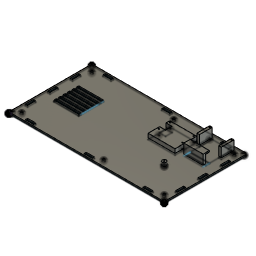
GBS 8200 Unterteil v2 (Autodesk Fusion 360 design; units mm, degrees)
Autodesk Fusion 360 part; units mm, degrees
sketch "Skizze1" plane through (0, 0, 0) normal (0, 1, 0) x (1, 0, 0)
  line L0 (2, 0) -> (206, 0)
  line L1 (208, 2) -> (208, 109)
  line L2 (206, 111) -> (2, 111)
  line L3 (0, 109) -> (0, 2)
  circle A0 centre (8.575, 8.575) radius 1.5
  circle A1 centre (8.575, 102.425) radius 1.5
  circle A2 centre (199.425, 102.425) radius 1.5
  circle A3 centre (199.425, 8.575) radius 1.5
  circle A4 centre (118.425, 8.575) radius 1.5
  circle A5 centre (118.425, 102.425) radius 1.5
  line L4 (123.425, 92.03) -> (159.425, 92.03)
  line L5 (159.425, 92.03) -> (159.425, 63.03)
  line L6 (159.425, 63.03) -> (123.425, 63.03)
  line L7 (123.425, 63.03) -> (123.425, 92.03)
  line L8 (123.425, 87.03) -> (131.425, 87.03)
  line L9 (131.425, 87.03) -> (131.425, 78.33)
  line L10 (131.425, 78.33) -> (123.425, 78.33)
  line L11 (123.425, 78.33) -> (123.425, 87.03)
  circle A6 centre (125.525, 90.23) radius 0.8
  circle A7 centre (157.325, 90.23) radius 0.8
  circle A8 centre (157.325, 75.23) radius 0.8
  circle A9 centre (125.525, 75.23) radius 0.8
  circle A10 centre (165.425, 42.575) radius 2.7
  circle A11 centre (165.425, 42.575) radius 0.8
  line L12 (166.2, 106) -> (192, 106)
  line L13 (192, 106) -> (192, 71.4)
  line L14 (192, 71.4) -> (166.2, 71.4)
  line L15 (166.2, 71.4) -> (166.2, 106)
  line L16 (166.2, 106) -> (162.8, 106)
  line L17 (162.8, 106) -> (162.8, 89)
  line L18 (162.8, 89) -> (166.2, 89)
  line L19 (166.2, 89) -> (166.2, 106)
  line L20 (192, 106) -> (195.4, 106)
  line L21 (195.4, 106) -> (195.4, 89)
  line L22 (195.4, 89) -> (192, 89)
  line L23 (192, 89) -> (192, 106)
  circle A12 centre (164.5, 104.3) radius 0.8
  circle A13 centre (193.7, 104.3) radius 0.8
  line L24 (166.2, 68) -> (192, 68)
  line L25 (192, 68) -> (192, 76.4)
  line L26 (192, 76.4) -> (166.2, 76.4)
  line L27 (166.2, 76.4) -> (166.2, 68)
  line L28 (166.2, 76.4) -> (192, 76.4)
  line L29 (192, 76.4) -> (192, 71.4)
  line L30 (192, 71.4) -> (166.2, 71.4)
  line L31 (166.2, 71.4) -> (166.2, 76.4)
  line L32 (16.5, 77) -> (49.5, 77)
  line L33 (49.5, 77) -> (49.5, 44)
  line L34 (49.5, 44) -> (16.5, 44)
  line L35 (16.5, 44) -> (16.5, 77)
  line L36 (16.5, 77) -> (49.5, 77)
  line L37 (49.5, 77) -> (49.5, 74)
  line L38 (49.5, 74) -> (16.5, 74)
  line L39 (16.5, 74) -> (16.5, 77)
  line L40 (16.5, 74) -> (49.5, 74)
  line L41 (49.5, 74) -> (49.5, 71)
  line L42 (49.5, 71) -> (16.5, 71)
  line L43 (16.5, 71) -> (16.5, 74)
  line L44 (16.5, 71) -> (49.5, 71)
  line L45 (49.5, 71) -> (49.5, 68)
  line L46 (49.5, 68) -> (16.5, 68)
  line L47 (16.5, 68) -> (16.5, 71)
  line L48 (16.5, 68) -> (49.5, 68)
  line L49 (49.5, 68) -> (49.5, 65)
  line L50 (49.5, 65) -> (16.5, 65)
  line L51 (16.5, 65) -> (16.5, 68)
  line L52 (16.5, 65) -> (49.5, 65)
  line L53 (49.5, 65) -> (49.5, 62)
  line L54 (49.5, 62) -> (16.5, 62)
  line L55 (16.5, 62) -> (16.5, 65)
  line L56 (16.5, 62) -> (49.5, 62)
  line L57 (49.5, 62) -> (49.5, 59)
  line L58 (49.5, 59) -> (16.5, 59)
  line L59 (16.5, 59) -> (16.5, 62)
  line L60 (16.5, 59) -> (49.5, 59)
  line L61 (49.5, 59) -> (49.5, 56)
  line L62 (49.5, 56) -> (16.5, 56)
  line L63 (16.5, 56) -> (16.5, 59)
  line L64 (16.5, 56) -> (49.5, 56)
  line L65 (49.5, 56) -> (49.5, 53)
  line L66 (49.5, 53) -> (16.5, 53)
  line L67 (16.5, 53) -> (16.5, 56)
  line L68 (16.5, 53) -> (49.5, 53)
  line L69 (49.5, 53) -> (49.5, 50)
  line L70 (49.5, 50) -> (16.5, 50)
  line L71 (16.5, 50) -> (16.5, 53)
  line L72 (16.5, 50) -> (49.5, 50)
  line L73 (49.5, 50) -> (49.5, 47)
  line L74 (49.5, 47) -> (16.5, 47)
  line L75 (16.5, 47) -> (16.5, 50)
  line L76 (16.5, 47) -> (49.5, 47)
  line L77 (49.5, 47) -> (49.5, 44)
  line L78 (49.5, 44) -> (16.5, 44)
  line L79 (16.5, 44) -> (16.5, 47)
  line L80 (20, 109) -> (30.8, 109)
  line L81 (30.8, 109) -> (30.8, 106)
  line L82 (30.8, 106) -> (20, 106)
  line L83 (20, 106) -> (20, 109)
  line L84 (2, 91) -> (5, 91)
  line L85 (5, 91) -> (5, 80.2)
  line L86 (5, 80.2) -> (2, 80.2)
  line L87 (2, 80.2) -> (2, 91)
  line L88 (2, 30.8) -> (5, 30.8)
  line L89 (5, 30.8) -> (5, 20)
  line L90 (5, 20) -> (2, 20)
  line L91 (2, 20) -> (2, 30.8)
  line L92 (20, 5) -> (30.8, 5)
  line L93 (30.8, 5) -> (30.8, 2)
  line L94 (30.8, 2) -> (20, 2)
  line L95 (20, 2) -> (20, 5)
  line L96 (177.2, 5) -> (188, 5)
  line L97 (188, 5) -> (188, 2)
  line L98 (188, 2) -> (177.2, 2)
  line L99 (177.2, 2) -> (177.2, 5)
  line L100 (203, 30.8) -> (206, 30.8)
  line L101 (206, 30.8) -> (206, 20)
  line L102 (206, 20) -> (203, 20)
  line L103 (203, 20) -> (203, 30.8)
  line L104 (177.2, 109) -> (188, 109)
  line L105 (188, 109) -> (188, 106)
  line L106 (188, 106) -> (177.2, 106)
  line L107 (177.2, 106) -> (177.2, 109)
  line L108 (203, 91) -> (206, 91)
  line L109 (206, 91) -> (206, 80.2)
  line L110 (206, 80.2) -> (203, 80.2)
  line L111 (203, 80.2) -> (203, 91)
  line L112 (98.6, 5) -> (109.4, 5)
  line L113 (109.4, 5) -> (109.4, 2)
  line L114 (109.4, 2) -> (98.6, 2)
  line L115 (98.6, 2) -> (98.6, 5)
  line L116 (98.6, 109) -> (109.4, 109)
  line L117 (109.4, 109) -> (109.4, 106)
  line L118 (109.4, 106) -> (98.6, 106)
  line L119 (98.6, 106) -> (98.6, 109)
  line L120 (203, 60.9) -> (206, 60.9)
  line L121 (206, 60.9) -> (206, 50.1)
  line L122 (206, 50.1) -> (203, 50.1)
  line L123 (203, 50.1) -> (203, 60.9)
  line L124 (2, 60.9) -> (5, 60.9)
  line L125 (5, 60.9) -> (5, 50.1)
  line L126 (5, 50.1) -> (2, 50.1)
  line L127 (2, 50.1) -> (2, 60.9)
  arc A14 (2, 111) -> (0, 109) centre (2, 109) ccw
  arc A15 (0, 2) -> (2, 0) centre (2, 2) ccw
  arc A16 (206, 0) -> (208, 2) centre (206, 2) ccw
  arc A17 (208, 109) -> (206, 111) centre (206, 109) ccw
  point P0 (208, 0)
  point P1 (0, 111)
  dimension "d1" = 208
  dimension "d2" = 111
  dimension "d3" = 3
  dimension "d4" = 8.575
  dimension "d5" = 8.575
  dimension "d6" = 3
  dimension "d7" = 8.575
  dimension "d8" = 8.575
  dimension "d9" = 3
  dimension "d10" = 8.575
  dimension "d11" = 8.575
  dimension "d12" = 3
  dimension "d13" = 8.575
  dimension "d14" = 8.575
  dimension "d15" = 3
  dimension "d16" = 8.575
  dimension "d17" = 109.85
  dimension "d18" = 3
  dimension "d19" = 8.575
  dimension "d20" = 109.85
  dimension "d21" = 36
  dimension "d22" = 29
  dimension "d23" = 18.97
  dimension "d24" = 5
  dimension "d25" = 5
  dimension "d26" = 8.7
  dimension "d27" = 8
  dimension "d28" = 1.6
  dimension "d29" = 1.6
  dimension "d30" = 31.8
  dimension "d31" = 2.1
  dimension "d32" = 1.8
  dimension "d33" = 1.8
  dimension "d34" = 1.6
  dimension "d35" = 2.1
  dimension "d36" = 15
  dimension "d37" = 1.6
  dimension "d38" = 15
  dimension "d39" = 2.1
  dimension "d40" = 5.4
  dimension "d41" = 34
  dimension "d42" = 34
  dimension "d43" = 1.6
  dimension "d44" = 25.8
  dimension "d45" = 34.6
  dimension "d46" = 5
  dimension "d47" = 16
  dimension "d48" = 3.4
  dimension "d49" = 3.4
  dimension "d50" = 17
  dimension "d51" = 17
  dimension "d52" = 1.6
  dimension "d53" = 1.7
  dimension "d54" = 1.7
  dimension "d55" = 1.6
  dimension "d56" = 1.7
  dimension "d57" = 1.7
  dimension "d58" = 8.4
  dimension "d59" = 5
  dimension "d60" = 33
  dimension "d61" = 33
  dimension "d62" = 34
  dimension "d63" = 16.5
  dimension "d64" = 3
  dimension "d65" = 33
  dimension "d66" = 3
  dimension "d67" = 3
  dimension "d68" = 3
  dimension "d69" = 3
  dimension "d70" = 3
  dimension "d71" = 3
  dimension "d72" = 3
  dimension "d73" = 3
  dimension "d74" = 3
  dimension "d75" = 10.8
  dimension "d76" = 3
  dimension "d77" = 20
  dimension "d78" = 2
  dimension "d79" = 3
  dimension "d80" = 10.8
  dimension "d81" = 2
  dimension "d82" = 20
  dimension "d83" = 3
  dimension "d84" = 10.8
  dimension "d85" = 2
  dimension "d86" = 20
  dimension "d87" = 10.8
  dimension "d88" = 3
  dimension "d89" = 2
  dimension "d90" = 20
  dimension "d91" = 10.8
  dimension "d92" = 3
  dimension "d93" = 2
  dimension "d94" = 20
  dimension "d95" = 3
  dimension "d96" = 10.8
  dimension "d97" = 2
  dimension "d98" = 20
  dimension "d99" = 10.8
  dimension "d100" = 3
  dimension "d101" = 2
  dimension "d102" = 20
  dimension "d103" = 3
  dimension "d104" = 10.8
  dimension "d105" = 2
  dimension "d106" = 20
  dimension "d107" = 10.8
  dimension "d108" = 3
  dimension "d109" = 2
  dimension "d110" = 98.6
  dimension "d111" = 10.8
  dimension "d112" = 3
  dimension "d113" = 2
  dimension "d114" = 98.6
  dimension "d115" = 3
  dimension "d116" = 10.8
  dimension "d117" = 2
  dimension "d118" = 50.1
  dimension "d119" = 3
  dimension "d120" = 10.8
  dimension "d121" = 2
  dimension "d122" = 50.1
  dimension "d123" = 2
  dimension "d124" = 2
  dimension "d125" = 2
  dimension "d126" = 2
  constraint horizontal L0
  constraint vertical L1
  constraint horizontal L2
  constraint vertical L3
  constraint horizontal L4
  constraint vertical L5
  constraint horizontal L6
  constraint vertical L7
  constraint horizontal L8
  constraint vertical L9
  constraint horizontal L10
  constraint vertical L11
  constraint coincident L7 L8.start
  constraint concentric A10 A11
  constraint horizontal L12
  constraint vertical L13
  constraint horizontal L14
  constraint vertical L15
  constraint horizontal L16
  constraint vertical L17
  constraint horizontal L18
  constraint vertical L19
  constraint horizontal L20
  constraint vertical L21
  constraint horizontal L22
  constraint vertical L23
  constraint horizontal L24
  constraint vertical L25
  constraint horizontal L26
  constraint vertical L27
  constraint horizontal L28
  constraint vertical L29
  constraint horizontal L30
  constraint vertical L31
  constraint horizontal L32
  constraint vertical L33
  constraint horizontal L34
  constraint vertical L35
  constraint horizontal L36
  constraint vertical L37
  constraint horizontal L38
  constraint vertical L39
  constraint horizontal L40
  constraint vertical L41
  constraint horizontal L42
  constraint vertical L43
  constraint horizontal L44
  constraint vertical L45
  constraint horizontal L46
  constraint vertical L47
  constraint horizontal L48
  constraint vertical L49
  constraint horizontal L50
  constraint vertical L51
  constraint horizontal L52
  constraint vertical L53
  constraint horizontal L54
  constraint vertical L55
  constraint horizontal L56
  constraint vertical L57
  constraint horizontal L58
  constraint vertical L59
  constraint horizontal L60
  constraint vertical L61
  constraint horizontal L62
  constraint vertical L63
  constraint horizontal L64
  constraint vertical L65
  constraint horizontal L66
  constraint vertical L67
  constraint horizontal L68
  constraint vertical L69
  constraint horizontal L70
  constraint vertical L71
  constraint horizontal L72
  constraint vertical L73
  constraint horizontal L74
  constraint vertical L75
  constraint horizontal L76
  constraint vertical L77
  constraint horizontal L78
  constraint vertical L79
  constraint horizontal L80
  constraint vertical L81
  constraint horizontal L82
  constraint vertical L83
  constraint horizontal L84
  constraint vertical L85
  constraint horizontal L86
  constraint vertical L87
  constraint horizontal L88
  constraint vertical L89
  constraint horizontal L90
  constraint vertical L91
  constraint horizontal L92
  constraint vertical L93
  constraint horizontal L94
  constraint vertical L95
  constraint horizontal L96
  constraint vertical L97
  constraint horizontal L98
  constraint vertical L99
  constraint horizontal L100
  constraint vertical L101
  constraint horizontal L102
  constraint vertical L103
  constraint horizontal L104
  constraint vertical L105
  constraint horizontal L106
  constraint vertical L107
  constraint horizontal L108
  constraint vertical L109
  constraint horizontal L110
  constraint vertical L111
  constraint horizontal L112
  constraint vertical L113
  constraint horizontal L114
  constraint vertical L115
  constraint horizontal L116
  constraint vertical L117
  constraint horizontal L118
  constraint vertical L119
  constraint horizontal L120
  constraint vertical L121
  constraint horizontal L122
  constraint vertical L123
  constraint horizontal L124
  constraint vertical L125
  constraint horizontal L126
  constraint vertical L127
  constraint coincident P1 L2
  constraint coincident P1 L3
  constraint tangent L2 A14
  constraint tangent L3 A14
  constraint coincident origin L3
  constraint coincident origin L0
  constraint tangent L3 A15
  constraint tangent L0 A15
  constraint coincident P0 L1
  constraint coincident P0 L0
  constraint tangent L1 A16
  constraint tangent L0 A16
  constraint tangent L2 A17
  constraint tangent L1 A17
  measures "d1" distance of origin P0
  measures "d2" distance of origin P1
  measures "d3" diameter of A0
  measures "d4" distance of L3 A0.centre
  measures "d5" distance of L0 A0.centre
  measures "d6" diameter of A1
  measures "d7" distance of L2 A1.centre
  measures "d8" distance of L3 A1.centre
  measures "d9" diameter of A2
  measures "d10" distance of L1 A2.centre
  measures "d11" distance of L2 A2.centre
  measures "d12" diameter of A3
  measures "d13" distance of L1 A3.centre
  measures "d14" distance of L0 A3.centre
  measures "d15" diameter of A4
  measures "d16" distance of L0 A4.centre
  measures "d17" distance of A0.centre A4.centre
  measures "d18" diameter of A5
  measures "d19" distance of L2 A5.centre
  measures "d20" distance of A1.centre A5.centre
  measures "d21" distance of L4.start L4.end
  measures "d22" distance of L4.start L6.end
  measures "d23" distance of L2 L4
  measures "d24" distance of A5.centre L7
  measures "d25" distance of L4 L8
  measures "d26" distance of L8.end L9.end
  measures "d27" distance of L9.end L10.end
  measures "d28" diameter of A6
  measures "d29" diameter of A7
  measures "d30" horizontal distance of A6.centre A7.centre
  measures "d31" distance of L5 A7.centre
  measures "d32" distance of L4 A6.centre
  measures "d33" distance of L4 A7.centre
  measures "d34" diameter of A8
  measures "d35" distance of L5 A8.centre
  measures "d36" distance of A7.centre A8.centre
  measures "d37" diameter of A9
  measures "d38" vertical distance of A6.centre A9.centre
  measures "d39" distance of L7 A9.centre
  measures "d40" diameter of A10
  measures "d41" horizontal distance of A3.centre A10.centre
  measures "d42" vertical distance of A3.centre A10.centre
  measures "d43" diameter of A11
  measures "d44" distance of L12.start L12.end
  measures "d45" distance of L12.start L14.end
  measures "d46" distance of L2 L12
  measures "d47" distance of L1 L13
  measures "d48" distance of L12.start L16.end
  measures "d49" distance of L12.end L20.end
  measures "d50" distance of L20.end L21.end
  measures "d51" distance of L12.start L18.end
  measures "d52" diameter of A12
  measures "d53" distance of L15 A12.centre
  measures "d54" distance of L16 A12.centre
  measures "d55" diameter of A13
  measures "d56" distance of L20 A13.centre
  measures "d57" distance of L21 A13.centre
  measures "d58" distance of L24.start L26.end
  measures "d59" distance of L14 L26
  measures "d60" distance of L32.start L32.end
  measures "d61" distance of L32.start L34.end
  measures "d62" distance of L2 L32
  measures "d63" distance of L3 L35
  measures "d64" distance of L32.start L38.end
  measures "d65" distance of L38.end L37.end
  measures "d66" distance of L38.end L42.end
  measures "d67" distance of L42.end L46.end
  measures "d68" distance of L46.end L50.end
  measures "d69" distance of L50.end L54.end
  measures "d70" distance of L54.end L58.end
  measures "d71" distance of L58.end L62.end
  measures "d72" distance of L62.end L66.end
  measures "d73" distance of L66.end L70.end
  measures "d74" distance of L70.end L74.end
  measures "d75" distance of L80.start L80.end
  measures "d76" distance of L80.start L82.end
  measures "d77" distance of L3 L83
  measures "d78" distance of L2 L80
  measures "d79" distance of L84.start L84.end
  measures "d80" distance of L84.start L86.end
  measures "d81" distance of L3 L87
  measures "d82" distance of L2 L84.end
  measures "d83" distance of L88.start L88.end
  measures "d84" distance of L88.start L90.end
  measures "d85" distance of L3 L91
  measures "d86" distance of L0 L90.end
  measures "d87" distance of L92.start L92.end
  measures "d88" distance of L92.start L94.end
  measures "d89" distance of L0 L93.end
  measures "d90" distance of L3 L92.start
  measures "d91" distance of L96.start L96.end
  measures "d92" distance of L96.start L98.end
  measures "d93" distance of L0 L97.end
  measures "d94" distance of L1 L97.end
  measures "d95" distance of L100.start L100.end
  measures "d96" distance of L100.start L102.end
  measures "d97" distance of L1 L101
  measures "d98" distance of L0 L102.end
  measures "d99" distance of L104.start L104.end
  measures "d100" distance of L104.start L106.end
  measures "d101" distance of L2 L104
  measures "d102" distance of L1 L105
  measures "d103" distance of L108.start L108.end
  measures "d104" distance of L108.start L110.end
  measures "d105" distance of L1 L109
  measures "d106" distance of L2 L108
  measures "d107" distance of L112.start L112.end
  measures "d108" distance of L112.start L114.end
  measures "d109" distance of L0 L114
  measures "d110" distance of L3 L114.end
  measures "d111" distance of L116.start L116.end
  measures "d112" distance of L116.start L118.end
  measures "d113" distance of L2 L116
  measures "d114" distance of L3 L118.end
  measures "d115" distance of L120.start L120.end
  measures "d116" distance of L120.start L122.end
  measures "d117" distance of L1 L121
  measures "d118" distance of L2 L120
  measures "d119" distance of L124.start L124.end
  measures "d120" distance of L124.start L126.end
  measures "d121" distance of L3 L127
  measures "d122" distance of L2 L124.end
  measures "d123" radius of A14
  measures "d124" radius of A15
  measures "d125" radius of A16
  measures "d126" radius of A17
extrude "Extrusion1" add sketch "Skizze1" along normal blind 1.8 contours L0 L1 L2 L3 A14 A15 A16 A17 | L12 L13 L15 L19 L23 L26 L28 L106 | L33 L35 L38 L40 L41 L42 L43 L44 | L33 L35 L46 L48 L49 L50 L51 L52 | L33 L35 L54 L56 L57 L58 L59 L60 | L33 L35 L62 L64 L65 L66 L67 L68 | L33 L35 L70 L72 L73 L74 L75 L76
extrude "Extrusion2" add sketch "Skizze1" along normal blind 1.8 contours L7 L8 L9 L10 L11
extrude "Extrusion3" add sketch "Skizze1" along normal blind 7.25 contours L4 L5 L6 L7 L8 L9 L10
extrude "Extrusion4" add sketch "Skizze1" along normal blind 14.1 contours L15 L16 L17 L18 L19 | L13 L20 L21 L22 L23
extrude "Extrusion5" add sketch "Skizze1" along normal blind 6.2 contours A10
extrude "Extrusion6" add sketch "Skizze1" along normal blind 14.8 contours L14 L24 L25 L27 L30
extrude "Extrusion7" add sketch "Skizze1" along normal blind 1.8 from surface at 13 contours L13 L14 L15 L25 L26 L27 L28 L29 L30 L31
extrude "Extrusion8" add sketch "Skizze1" along normal blind 1.8 contours L13 L14 L15 L25 L26 L27 L28 L29 L30 L31
